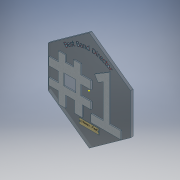
# Autodesk Inventor part: Trophy
Saved by Autodesk Inventor 2018 (Build 220112000, 112)
## iProperties
Created: 2019-03-04
Part Number: Trophy
Material: Generic
Document SubType Name: Modeling
Designer: This kid
Density: 1 g/cm^3
Appearance: Expanded Metal 01
Author: This kid
Autodesk Inventor part; units mm, degrees
(part 1 of 3)
ref_plane "YZ Plane" through (0, 0, 0) normal (1, 0, 0) x (0, 1, 0)
ref_plane "XZ Plane" through (0, 0, 0) normal (0, 1, 0) x (-1, 0, 0)
ref_plane "XY Plane" through (0, 0, 0) normal (0, 0, 1) x (1, 0, 0)
sketch "Sketch1" plane through (0, 0, 0) normal (0, 0, 1) x (1, 0, 0)
  line L0 (4871.8502, -2409.9611) -> (4871.8502, 2409.9611)
  line L1 (-4871.8502, 2409.9611) -> (-4871.8502, -2409.9611)
  line L2 (-4871.8502, 2409.9611) -> (0, 5903.7537)
  line L3 (0, 5903.7537) -> (4871.8502, 2409.9611)
  line L4 (-4871.8502, -2409.9611) -> (0, -5895.763)
  line L5 (0, -5895.763) -> (4871.8502, -2409.9611)
  point P0 (0, 0)
  constraints: 12 end point, 1 parallel
extrude "Extrusion1" add sketch "Sketch1" along normal blind 304.8
sketch "Sketch5" plane through (0, 0, 304.8) normal (0, 0, 1) x (1, 0, 0)
  line L0 (-1178.5841, -3968.2328) -> (1176.6192, -3968.2328)
  line L1 (1176.6192, -3968.2328) -> (1176.6192, -3311.2191)
  line L2 (1176.6192, -3311.2191) -> (-1178.5841, -3311.2191)
  line L3 (-1178.5841, -3311.2191) -> (-1178.5841, -3968.2328)
  line L4 (-1178.5841, -3968.2328) -> (1176.6192, -3311.2191) construction
  line L5 (1176.6192, -3968.2328) -> (-1178.5841, -3311.2191) construction
  point P0 (0, 0)
  point P1 (-0.9824, -3639.7259)
  constraints: 12 end point, 2 midpoint, 2 parallel, 1 horizontal, 1 perpendicular
extrude "Extrusion2" add sketch "Sketch5" along normal blind 25.4
sketch "Sketch6" plane through (0, 0, 330.2) normal (0, 0, 1) x (1, 0, 0)
  point P0 (0, 0)
sketch "Sketch7" plane through (0, 0, 330.2) normal (0, 0, 1) x (1, 0, 0)
  line L0 (-1178.5841, -3311.2191) -> (1176.6192, -3311.2191) construction
  line L1 (-0.9824, -3311.2191) -> (-0.9824, -3968.2328) construction
  line L2 (1176.6192, -3968.2328) -> (-1178.5841, -3968.2328) construction
  line L3 (-1178.5841, -3968.2328) -> (-1178.5841, -3311.2191) construction
  line L4 (-1178.5841, -3639.7259) -> (1176.6192, -3639.7259) construction
  line L5 (1176.6192, -3311.2191) -> (1176.6192, -3968.2328) construction
  line L6 (1176.6192, -3490.7913) -> (1021.494, -3490.7913) construction
  line L7 (-1178.5841, -3918.298) -> (-1023.4589, -3918.298) construction
  line L8 (-1101.0215, -3918.298) -> (-1101.0215, -3968.2328)
  line L9 (-1101.0215, -3311.2191) -> (-1101.0215, -3918.298)
  line L10 (1099.0566, -3490.7913) -> (1099.0566, -3311.2191)
  line L11 (1099.0566, -3968.2328) -> (1099.0566, -3490.7913)
  point P0 (0, 0)
  point P1 (-1023.4589, -3439.1683)
  point P2 (1110.7745, -3639.7259)
  point P3 (-1101.0215, -3639.7259)
  point P4 (1099.0566, -3639.7259)
  constraints: 16 end point, 12 point on line, 6 midpoint, 2 collinear, 2 perpendicular, 1 horizontal, 1 parallel
sketch "Sketch8" plane through (0, 0, 330.2) normal (0, 0, 1) x (1, 0, 0)
  line L0 (-1188.8601, -3420.1858) -> (1172.5443, -3420.1858) construction
  line L1 (1172.5443, -3420.1858) -> (1172.5443, -3747.7413) construction
  line L2 (1172.5443, -3747.7413) -> (-1188.8601, -3747.7413) construction
  line L3 (-1188.8601, -3747.7413) -> (-1188.8601, -3420.1858) construction
  point P0 (0, 0)
  constraints: 2 other
sketch "Sketch9" plane through (0, 0, 304.8) normal (0, 0, 1) x (1, 0, 0)
  arc A0 (3785.7257, 1434.029) -> (-2757.9123, 2963.4571) centre (0, 0) ccw construction
  spline S0 degree 2 poles (-2558.5983, 3341.4787) (-2534.2376, 3312.4793) (-2518.9668, 3249.4993) (-2525.0687, 3219.6418) knots 0 0 0 1 2 2 2
  spline S1 degree 2 poles (-2525.0687, 3219.6418) (-2532.8347, 3184.0851) (-2570.7728, 3127.4837) (-2610.4893, 3094.1201) knots 0 0 0 1 2 2 2
  line L0 (-2610.4893, 3094.1201) -> (-2722.0737, 3000.3842)
  line L1 (-2722.0737, 3000.3842) -> (-3048.8254, 3389.3537)
  line L2 (-3048.8254, 3389.3537) -> (-2945.7517, 3475.9402)
  spline S2 degree 2 poles (-2945.7517, 3475.9402) (-2904.1439, 3510.8926) (-2858.0347, 3540.4864) (-2830.384, 3545.9719) knots 0 0 0 1 2 2 2
  spline S3 degree 2 poles (-2830.384, 3545.9719) (-2799.9972, 3552.6805) (-2750.3185, 3532.5836) (-2729.6648, 3507.9972) knots 0 0 0 1 2 2 2
  spline S4 degree 2 poles (-2729.6648, 3507.9972) (-2706.628, 3480.5739) (-2699.0862, 3412.7141) (-2714.2914, 3378.9729) knots 0 0 0 1 2 2 2
  line L3 (-2714.2914, 3378.9729) -> (-2712.7027, 3377.0816)
  spline S5 degree 2 poles (-2712.7027, 3377.0816) (-2670.0858, 3396.7523) (-2589.8437, 3378.6735) (-2558.5983, 3341.4787) knots 0 0 0 1 2 2 2
  spline S6 degree 2 poles (-2610.6458, 3293.993) (-2629.1811, 3316.0577) (-2665.6207, 3333.835) (-2693.0066, 3328.0343) knots 0 0 0 1 2 2 2
  spline S7 degree 2 poles (-2693.0066, 3328.0343) (-2710.5956, 3324.0117) (-2742.7725, 3303.4335) (-2769.5654, 3280.9263) knots 0 0 0 1 2 2 2
  line L4 (-2769.5654, 3280.9263) -> (-2828.1945, 3231.6752)
  line L5 (-2828.1945, 3231.6752) -> (-2707.4499, 3087.9393)
  line L6 (-2707.4499, 3087.9393) -> (-2665.5269, 3123.1564)
  spline S8 degree 2 poles (-2665.5269, 3123.1564) (-2631.4842, 3151.7538) (-2597.694, 3190.8921) (-2591.0372, 3213.6888) knots 0 0 0 1 2 2 2
  spline S9 degree 2 poles (-2591.0372, 3213.6888) (-2585.2756, 3236.2711) (-2593.4344, 3273.5043) (-2610.6458, 3293.993) knots 0 0 0 1 2 2 2
  spline S10 degree 2 poles (-2777.4756, 3455.4681) (-2789.1264, 3469.3374) (-2816.0589, 3482.1975) (-2831.4918, 3479.4484) knots 0 0 0 1 2 2 2
  spline S11 degree 2 poles (-2831.4918, 3479.4484) (-2849.9256, 3475.7914) (-2883.1489, 3453.2589) (-2910.5722, 3430.2221) knots 0 0 0 1 2 2 2
  line L7 (-2910.5722, 3430.2221) -> (-2960.0602, 3388.6499)
  line L8 (-2960.0602, 3388.6499) -> (-2864.4708, 3274.859)
  line L9 (-2864.4708, 3274.859) -> (-2805.8417, 3324.1101)
  spline S12 degree 2 poles (-2805.8417, 3324.1101) (-2781.5705, 3344.499) (-2762.7968, 3368.872) (-2757.1234, 3387.0791) knots 0 0 0 1 2 2 2
  spline S13 degree 2 poles (-2757.1234, 3387.0791) (-2751.5003, 3404.7062) (-2762.1177, 3437.1859) (-2777.4756, 3455.4681) knots 0 0 0 1 2 2 2
  spline S14 degree 2 poles (-2266.0484, 3344.2576) (-2341.3465, 3292.4654) (-2482.1979, 3319.9967) (-2535.8564, 3398.0083) knots 0 0 0 1 2 2 2
  spline S15 degree 2 poles (-2535.8564, 3398.0083) (-2588.5818, 3474.6632) (-2570.7199, 3620.8553) (-2505.9363, 3665.4152) knots 0 0 0 1 2 2 2
  spline S16 degree 2 poles (-2505.9363, 3665.4152) (-2476.7668, 3685.4789) (-2419.9908, 3699.5485) (-2391.0061, 3693.0035) knots 0 0 0 1 2 2 2
  spline S17 degree 2 poles (-2391.0061, 3693.0035) (-2361.6823, 3686.6918) (-2308.0111, 3647.1619) (-2282.115, 3609.5129) knots 0 0 0 1 2 2 2
  line L10 (-2282.115, 3609.5129) -> (-2262.2847, 3580.6825)
  line L11 (-2262.2847, 3580.6825) -> (-2479.6996, 3431.1384)
  spline S18 degree 2 poles (-2479.6996, 3431.1384) (-2442.1386, 3376.5303) (-2347.2973, 3356.3247) (-2298.4553, 3389.9196) knots 0 0 0 1 2 2 2
  spline S19 degree 2 poles (-2298.4553, 3389.9196) (-2281.157, 3401.8178) (-2252.944, 3432.7155) (-2243.5761, 3448.1526) knots 0 0 0 1 2 2 2
  spline S20 degree 2 poles (-2243.5761, 3448.1526) (-2233.9965, 3464.7348) (-2222.4894, 3490.1374) (-2219.7778, 3499.997) knots 0 0 0 1 2 2 2
  line L12 (-2219.7778, 3499.997) -> (-2216.7252, 3502.0966)
  line L13 (-2216.7252, 3502.0966) -> (-2177.0645, 3444.4359)
  spline S21 degree 2 poles (-2177.0645, 3444.4359) (-2183.6561, 3434.4059) (-2204.0034, 3404.4216) (-2212.7575, 3393.9035) knots 0 0 0 1 2 2 2
  spline S22 degree 2 poles (-2212.7575, 3393.9035) (-2224.9877, 3378.9957) (-2247.0542, 3357.3223) (-2266.0484, 3344.2576) knots 0 0 0 1 2 2 2
  spline S23 degree 2 poles (-2341.6026, 3585.5837) (-2356.9788, 3606.4855) (-2387.2609, 3631.6244) (-2402.9727, 3636.3065) knots 0 0 0 1 2 2 2
  spline S24 degree 2 poles (-2402.9727, 3636.3065) (-2420.296, 3641.8788) (-2457.7584, 3634.5982) (-2479.1268, 3619.9004) knots 0 0 0 1 2 2 2
  spline S25 degree 2 poles (-2479.1268, 3619.9004) (-2500.156, 3605.4359) (-2521.0327, 3572.5893) (-2524.8445, 3551.98) knots 0 0 0 1 2 2 2
  spline S26 degree 2 poles (-2524.8445, 3551.98) (-2528.0838, 3531.2649) (-2519.5307, 3492.6791) (-2507.4621, 3471.5009) knots 0 0 0 1 2 2 2
  line L14 (-2507.4621, 3471.5009) -> (-2341.6026, 3585.5837)
  spline S27 degree 2 poles (-2007.8449, 3504.7842) (-2041.0949, 3485.8054) (-2108.8605, 3470.826) (-2133.5235, 3470.0209) knots 0 0 0 1 2 2 2
  line L15 (-2133.5235, 3470.0209) -> (-2169.2363, 3532.5882)
  line L16 (-2169.2363, 3532.5882) -> (-2166.3761, 3534.2208)
  spline S28 degree 2 poles (-2166.3761, 3534.2208) (-2155.9604, 3532.5818) (-2128.8991, 3530.0157) (-2108.5248, 3531.6909) knots 0 0 0 1 2 2 2
  spline S29 degree 2 poles (-2108.5248, 3531.6909) (-2090.7039, 3532.8568) (-2050.6672, 3542.437) (-2032.4333, 3552.8448) knots 0 0 0 1 2 2 2
  spline S30 degree 2 poles (-2032.4333, 3552.8448) (-2019.2048, 3560.3955) (-1992.2842, 3583.8197) (-1987.9907, 3592.9065) knots 0 0 0 1 2 2 2
  spline S31 degree 2 poles (-1987.9907, 3592.9065) (-1981.4998, 3605.6177) (-1980.9792, 3626.2972) (-1989.9585, 3642.0284) knots 0 0 0 1 2 2 2
  spline S32 degree 2 poles (-1989.9585, 3642.0284) (-2001.1825, 3661.6924) (-2034.2663, 3669.8271) (-2065.6733, 3660.9065) knots 0 0 0 1 2 2 2
  spline S33 degree 2 poles (-2065.6733, 3660.9065) (-2077.8276, 3657.287) (-2116.2317, 3644.8465) (-2133.1351, 3640.4123) knots 0 0 0 1 2 2 2
  spline S34 degree 2 poles (-2133.1351, 3640.4123) (-2177.3593, 3629.8639) (-2237.8033, 3656.0363) (-2256.374, 3688.5713) knots 0 0 0 1 2 2 2
  spline S35 degree 2 poles (-2256.374, 3688.5713) (-2282.0872, 3733.6198) (-2246.554, 3828.3214) (-2190.7798, 3860.1568) knots 0 0 0 1 2 2 2
  spline S36 degree 2 poles (-2190.7798, 3860.1568) (-2163.2502, 3875.8705) (-2099.7211, 3894.1198) (-2074.854, 3894.5674) knots 0 0 0 1 2 2 2
  line L17 (-2074.854, 3894.5674) -> (-2040.7738, 3834.8604)
  line L18 (-2040.7738, 3834.8604) -> (-2043.634, 3833.2278)
  spline S37 degree 2 poles (-2043.634, 3833.2278) (-2074.8812, 3838.1447) (-2138.3042, 3828.014) (-2165.1188, 3812.7085) knots 0 0 0 1 2 2 2
  spline S38 degree 2 poles (-2165.1188, 3812.7085) (-2192.6484, 3796.9949) (-2217.2815, 3752.1239) (-2204.0167, 3728.8846) knots 0 0 0 1 2 2 2
  spline S39 degree 2 poles (-2204.0167, 3728.8846) (-2191.9764, 3707.7905) (-2157.82, 3700.268) (-2129.1198, 3708.1177) knots 0 0 0 1 2 2 2
  spline S40 degree 2 poles (-2129.1198, 3708.1177) (-2115.1272, 3711.8384) (-2080.7065, 3722.9532) (-2061.6579, 3728.6118) knots 0 0 0 1 2 2 2
  spline S41 degree 2 poles (-2061.6579, 3728.6118) (-2019.8843, 3740.1316) (-1958.4167, 3718.8095) (-1937.3972, 3681.9842) knots 0 0 0 1 2 2 2
  spline S42 degree 2 poles (-1937.3972, 3681.9842) (-1925.1528, 3660.5325) (-1920.3248, 3613.0432) (-1928.8122, 3589.7122) knots 0 0 0 1 2 2 2
  spline S43 degree 2 poles (-1928.8122, 3589.7122) (-1937.964, 3565.054) (-1973.8798, 3524.1712) (-2007.8449, 3504.7842) knots 0 0 0 1 2 2 2
  spline S44 degree 2 poles (-1722.0451, 3655.7889) (-1769.0922, 3632.9858) (-1848.1015, 3661.0251) (-1876.2911, 3719.1856) knots 0 0 0 1 2 2 2
  line L19 (-1876.2911, 3719.1856) -> (-1968.4012, 3909.2262)
  line L20 (-1968.4012, 3909.2262) -> (-2007.2984, 3890.3733)
  line L21 (-2007.2984, 3890.3733) -> (-2030.4605, 3938.1613)
  line L22 (-2030.4605, 3938.1613) -> (-1991.5633, 3957.0142)
  line L23 (-1991.5633, 3957.0142) -> (-2039.3241, 4055.5538)
  line L24 (-2039.3241, 4055.5538) -> (-1981.534, 4083.5639)
  line L25 (-1981.534, 4083.5639) -> (-1933.7732, 3985.0243)
  line L26 (-1933.7732, 3985.0243) -> (-1827.4542, 4036.5556)
  line L27 (-1827.4542, 4036.5556) -> (-1804.292, 3988.7677)
  line L28 (-1804.292, 3988.7677) -> (-1910.611, 3937.2363)
  line L29 (-1910.611, 3937.2363) -> (-1831.4287, 3773.8681)
  spline S45 degree 2 poles (-1831.4287, 3773.8681) (-1818.8601, 3747.9366) (-1803.1824, 3720.3098) (-1790.9595, 3711.1373) knots 0 0 0 1 2 2 2
  spline S46 degree 2 poles (-1790.9595, 3711.1373) (-1780.5662, 3702.908) (-1752.0209, 3703.4767) (-1732.0166, 3713.1725) knots 0 0 0 1 2 2 2
  spline S47 degree 2 poles (-1732.0166, 3713.1725) (-1717.9396, 3719.9955) (-1695.7673, 3741.264) (-1691.097, 3746.73) knots 0 0 0 1 2 2 2
  line L30 (-1691.097, 3746.73) -> (-1687.763, 3748.3459)
  line L31 (-1687.763, 3748.3459) -> (-1662.6257, 3696.483)
  spline S48 degree 2 poles (-1662.6257, 3696.483) (-1676.7709, 3684.1373) (-1707.5976, 3662.7914) (-1722.0451, 3655.7889) knots 0 0 0 1 2 2 2
  spline S49 degree 2 poles (-1132.9212, 4053.1956) (-1121.0879, 4017.2181) (-1130.3262, 3953.0751) (-1147.0909, 3927.6262) knots 0 0 0 1 2 2 2
  spline S50 degree 2 poles (-1147.0909, 3927.6262) (-1167.5195, 3897.5053) (-1223.7813, 3859.0655) (-1273.0548, 3842.8589) knots 0 0 0 1 2 2 2
  line L32 (-1273.0548, 3842.8589) -> (-1411.4899, 3797.3262)
  line L33 (-1411.4899, 3797.3262) -> (-1570.2112, 4279.8939)
  line L34 (-1570.2112, 4279.8939) -> (-1442.3347, 4321.9537)
  spline S51 degree 2 poles (-1442.3347, 4321.9537) (-1390.7148, 4338.932) (-1336.9083, 4349.2623) (-1309.2002, 4344.0747) knots 0 0 0 1 2 2 2
  spline S52 degree 2 poles (-1309.2002, 4344.0747) (-1278.4973, 4339.0054) (-1239.851, 4301.8796) (-1229.8184, 4271.3769) knots 0 0 0 1 2 2 2
  spline S53 degree 2 poles (-1229.8184, 4271.3769) (-1218.6282, 4237.3547) (-1236.8556, 4171.5551) (-1263.5151, 4145.8853) knots 0 0 0 1 2 2 2
  line L35 (-1263.5151, 4145.8853) -> (-1262.7434, 4143.539)
  spline S54 degree 2 poles (-1262.7434, 4143.539) (-1215.8681, 4145.9557) (-1148.0988, 4099.3407) (-1132.9212, 4053.1956) knots 0 0 0 1 2 2 2
  spline S55 degree 2 poles (-1198.8921, 4028.4636) (-1207.8957, 4055.8378) (-1235.1142, 4085.8882) (-1262.6937, 4090.6847) knots 0 0 0 1 2 2 2
  spline S56 degree 2 poles (-1262.6937, 4090.6847) (-1280.5175, 4093.4896) (-1318.0385, 4086.349) (-1351.2786, 4075.416) knots 0 0 0 1 2 2 2
  line L36 (-1351.2786, 4075.416) -> (-1424.0157, 4051.492)
  line L37 (-1424.0157, 4051.492) -> (-1365.3634, 3873.1688)
  line L38 (-1365.3634, 3873.1688) -> (-1313.3525, 3890.2757)
  spline S57 degree 2 poles (-1313.3525, 3890.2757) (-1271.118, 3904.1671) (-1225.1991, 3927.9376) (-1210.5442, 3946.6254) knots 0 0 0 1 2 2 2
  spline S58 degree 2 poles (-1210.5442, 3946.6254) (-1196.8, 3965.447) (-1190.5316, 4003.0447) (-1198.8921, 4028.4636) knots 0 0 0 1 2 2 2
  spline S59 degree 2 poles (-1293.7313, 4240.3879) (-1299.3907, 4257.5946) (-1319.6116, 4279.5458) (-1334.9604, 4282.7314) knots 0 0 0 1 2 2 2
  spline S60 degree 2 poles (-1334.9604, 4282.7314) (-1353.4325, 4286.1898) (-1392.6516, 4277.6239) (-1426.6738, 4266.4336) knots 0 0 0 1 2 2 2
  line L39 (-1426.6738, 4266.4336) -> (-1488.0701, 4246.2398)
  line L40 (-1488.0701, 4246.2398) -> (-1441.6371, 4105.0672)
  line L41 (-1441.6371, 4105.0672) -> (-1368.9, 4128.9912)
  spline S61 degree 2 poles (-1368.9, 4128.9912) (-1338.7884, 4138.8952) (-1312.299, 4154.5416) (-1300.2633, 4169.3344) knots 0 0 0 1 2 2 2
  spline S62 degree 2 poles (-1300.2633, 4169.3344) (-1288.49, 4183.6076) (-1286.2711, 4217.7065) (-1293.7313, 4240.3879) knots 0 0 0 1 2 2 2
  spline S63 degree 2 poles (-825.2961, 4005.1241) (-831.6592, 3997.7819) (-852.8354, 3971.9091) (-863.5255, 3963.1697) knots 0 0 0 1 2 2 2
  spline S64 degree 2 poles (-863.5255, 3963.1697) (-877.9995, 3950.6234) (-906.8404, 3934.4169) (-934.952, 3928.0807) knots 0 0 0 1 2 2 2
  spline S65 degree 2 poles (-934.952, 3928.0807) (-957.8429, 3922.9212) (-1003.0994, 3930.8665) (-1022.2918, 3942.9985) knots 0 0 0 1 2 2 2
  spline S66 degree 2 poles (-1022.2918, 3942.9985) (-1040.5904, 3954.91) (-1068.8001, 3995.8153) (-1074.4122, 4020.7142) knots 0 0 0 1 2 2 2
  spline S67 degree 2 poles (-1074.4122, 4020.7142) (-1083.1018, 4059.2673) (-1062.883, 4121.2161) (-1031.0728, 4144.8438) knots 0 0 0 1 2 2 2
  spline S68 degree 2 poles (-1031.0728, 4144.8438) (-1003.007, 4166.3615) (-920.3129, 4196.3942) (-871.5504, 4210.339) knots 0 0 0 1 2 2 2
  line L42 (-871.5504, 4210.339) -> (-874.2659, 4222.3868)
  spline S69 degree 2 poles (-874.2659, 4222.3868) (-879.1539, 4244.0729) (-898.4711, 4267.9927) (-912.2388, 4272.9075) knots 0 0 0 1 2 2 2
  spline S70 degree 2 poles (-912.2388, 4272.9075) (-926.0065, 4277.8223) (-961.6298, 4274.8569) (-980.1032, 4270.6932) knots 0 0 0 1 2 2 2
  spline S71 degree 2 poles (-980.1032, 4270.6932) (-1001.7893, 4265.8052) (-1057.5256, 4239.7387) (-1084.0359, 4220.6815) knots 0 0 0 1 2 2 2
  line L43 (-1084.0359, 4220.6815) -> (-1087.6503, 4219.8668)
  line L44 (-1087.6503, 4219.8668) -> (-1102.0425, 4283.7204)
  spline S72 degree 2 poles (-1102.0425, 4283.7204) (-1085.8602, 4292.4318) (-1023.9189, 4319.0529) (-992.193, 4326.2037) knots 0 0 0 1 2 2 2
  spline S73 degree 2 poles (-992.193, 4326.2037) (-953.6399, 4334.8934) (-898.3154, 4334.7033) (-873.9023, 4323.748) knots 0 0 0 1 2 2 2
  spline S74 degree 2 poles (-873.9023, 4323.748) (-849.9814, 4313.1038) (-818.949, 4269.0367) (-811.0741, 4234.0979) knots 0 0 0 1 2 2 2
  line L45 (-811.0741, 4234.0979) -> (-753.7767, 3979.8885)
  line L46 (-753.7767, 3979.8885) -> (-816.4254, 3965.7678)
  line L47 (-816.4254, 3965.7678) -> (-825.2961, 4005.1241)
  line L48 (-837.0634, 4057.3314) -> (-860.3263, 4160.5412)
  spline S75 degree 2 poles (-860.3263, 4160.5412) (-882.363, 4153.4643) (-948.6937, 4131.3398) (-968.53, 4120.1169) knots 0 0 0 1 2 2 2
  spline S76 degree 2 poles (-968.53, 4120.1169) (-991.709, 4106.8745) (-1017.0873, 4067.8166) (-1010.7511, 4039.705) knots 0 0 0 1 2 2 2
  spline S77 degree 2 poles (-1010.7511, 4039.705) (-1003.5097, 4007.5774) (-960.0343, 3983.1948) (-925.4972, 3990.9793) knots 0 0 0 1 2 2 2
  spline S78 degree 2 poles (-925.4972, 3990.9793) (-896.1808, 3997.587) (-853.692, 4033.7496) (-837.0634, 4057.3314) knots 0 0 0 1 2 2 2
  line L49 (-368.3427, 4034.2667) -> (-432.0348, 4026.0464)
  line L50 (-432.0348, 4026.0464) -> (-459.8575, 4241.6198)
  spline S79 degree 2 poles (-459.8575, 4241.6198) (-463.23, 4267.7499) (-473.9258, 4312.0286) (-483.0138, 4324.5535) knots 0 0 0 1 2 2 2
  spline S80 degree 2 poles (-483.0138, 4324.5535) (-492.6155, 4337.8422) (-522.1704, 4348.1406) (-545.8508, 4345.0843) knots 0 0 0 1 2 2 2
  spline S81 degree 2 poles (-545.8508, 4345.0843) (-569.5312, 4342.028) (-616.4829, 4310.233) (-637.9369, 4286.7099) knots 0 0 0 1 2 2 2
  line L51 (-637.9369, 4286.7099) -> (-601.4722, 4004.1781)
  line L52 (-601.4722, 4004.1781) -> (-665.1643, 3995.9577)
  line L53 (-665.1643, 3995.9577) -> (-713.9596, 4374.0277)
  line L54 (-713.9596, 4374.0277) -> (-650.2674, 4382.2481)
  line L55 (-650.2674, 4382.2481) -> (-644.8399, 4340.1949)
  spline S82 degree 2 poles (-644.8399, 4340.1949) (-619.5798, 4369.6054) (-567.9395, 4403.6658) (-536.91, 4407.6706) knots 0 0 0 1 2 2 2
  spline S83 degree 2 poles (-536.91, 4407.6706) (-481.3835, 4414.8371) (-409.0229, 4349.4611) (-400.0121, 4279.6448) knots 0 0 0 1 2 2 2
  line L56 (-400.0121, 4279.6448) -> (-368.3427, 4034.2667)
  line L57 (14.388, 4050.8554) -> (-49.7982, 4048.76)
  line L58 (-49.7982, 4048.76) -> (-51.0608, 4087.4363)
  spline S84 degree 2 poles (-51.0608, 4087.4363) (-65.4701, 4074.6092) (-86.7396, 4057.4393) (-101.3235, 4049.9611) knots 0 0 0 1 2 2 2
  spline S85 degree 2 poles (-101.3235, 4049.9611) (-114.6864, 4042.9346) (-143.6711, 4034.9863) (-163.0092, 4034.355) knots 0 0 0 1 2 2 2
  spline S86 degree 2 poles (-163.0092, 4034.355) (-194.2794, 4033.3341) (-247.7913, 4057.5362) (-267.1259, 4082.0302) knots 0 0 0 1 2 2 2
  spline S87 degree 2 poles (-267.1259, 4082.0302) (-286.4605, 4106.5242) (-309.4508, 4179.9136) (-311.0224, 4228.0533) knots 0 0 0 1 2 2 2
  spline S88 degree 2 poles (-311.0224, 4228.0533) (-312.6611, 4278.2502) (-289.1307, 4352.3346) (-267.4009, 4380.6405) knots 0 0 0 1 2 2 2
  spline S89 degree 2 poles (-267.4009, 4380.6405) (-247.2229, 4406.0126) (-189.3123, 4436.3234) (-156.8078, 4437.3846) knots 0 0 0 1 2 2 2
  spline S90 degree 2 poles (-156.8078, 4437.3846) (-128.4177, 4438.3114) (-85.6219, 4426.9399) (-61.7394, 4414.5392) knots 0 0 0 1 2 2 2
  line L59 (-61.7394, 4414.5392) -> (-67.1123, 4579.1192)
  line L60 (-67.1123, 4579.1192) -> (-2.9261, 4581.2147)
  line L61 (-2.9261, 4581.2147) -> (14.388, 4050.8554)
  line L62 (-52.8205, 4141.3363) -> (-60.0067, 4361.4621)
  spline S91 degree 2 poles (-60.0067, 4361.4621) (-84.2469, 4372.2036) (-122.3824, 4379.6083) (-144.1892, 4378.8964) knots 0 0 0 1 2 2 2
  spline S92 degree 2 poles (-144.1892, 4378.8964) (-193.5633, 4377.2846) (-247.1027, 4301.3968) (-244.8192, 4231.4502) knots 0 0 0 1 2 2 2
  spline S93 degree 2 poles (-244.8192, 4231.4502) (-242.6163, 4163.9724) (-197.5017, 4094.1885) (-150.185, 4095.7332) knots 0 0 0 1 2 2 2
  spline S94 degree 2 poles (-150.185, 4095.7332) (-125.0865, 4096.5525) (-74.8189, 4121.2593) (-52.8205, 4141.3363) knots 0 0 0 1 2 2 2
  spline S95 degree 2 poles (759.7655, 4239.6528) (750.9285, 4170.6442) (680.7638, 4066.7408) (629.8313, 4041.7206) knots 0 0 0 1 2 2 2
  spline S96 degree 2 poles (629.8313, 4041.7206) (588.3627, 4022.5441) (507.4625, 4016.3026) (446.2122, 4024.146) knots 0 0 0 1 2 2 2
  line L63 (446.2122, 4024.146) -> (330.2451, 4038.9963)
  line L64 (330.2451, 4038.9963) -> (394.7705, 4542.8816)
  line L65 (394.7705, 4542.8816) -> (509.5126, 4528.1883)
  spline S97 degree 2 poles (509.5126, 4528.1883) (580.5629, 4519.0899) (658.6942, 4487.5031) (684.8723, 4465.0594) knots 0 0 0 1 2 2 2
  spline S98 degree 2 poles (684.8723, 4465.0594) (729.3333, 4426.5785) (769.1776, 4313.1531) (759.7655, 4239.6528) knots 0 0 0 1 2 2 2
  spline S99 degree 2 poles (690.0448, 4249.411) (697.4699, 4307.3946) (669.5966, 4394.3851) (634.602, 4422.5232) knots 0 0 0 1 2 2 2
  spline S100 degree 2 poles (634.602, 4422.5232) (609.6911, 4441.8993) (550.6794, 4463.9822) (505.3542, 4469.7864) knots 0 0 0 1 2 2 2
  line L66 (505.3542, 4469.7864) -> (454.3123, 4476.3226)
  line L67 (454.3123, 4476.3226) -> (404.6372, 4088.4043)
  line L68 (404.6372, 4088.4043) -> (455.679, 4081.8681)
  spline S101 degree 2 poles (455.679, 4081.8681) (500.1876, 4076.1686) (569.393, 4081.8325) (599.209, 4097.5208) knots 0 0 0 1 2 2 2
  spline S102 degree 2 poles (599.209, 4097.5208) (637.3586, 4116.7074) (682.515, 4190.6108) (690.0448, 4249.411) knots 0 0 0 1 2 2 2
  line L69 (857.6796, 3956.4599) -> (794.811, 3969.5673)
  line L70 (794.811, 3969.5673) -> (872.6153, 4342.7488)
  line L71 (872.6153, 4342.7488) -> (935.4839, 4329.6414)
  line L72 (935.4839, 4329.6414) -> (857.6796, 3956.4599)
  line L73 (952.8563, 4390.7797) -> (881.5246, 4405.6516)
  line L74 (881.5246, 4405.6516) -> (895.1362, 4470.9382)
  line L75 (895.1362, 4470.9382) -> (966.4678, 4456.0663)
  line L76 (966.4678, 4456.0663) -> (952.8563, 4390.7797)
  line L77 (1224.4433, 4187.0481) -> (1221.2576, 4187.8832)
  spline S103 degree 2 poles (1221.2576, 4187.8832) (1214.6117, 4191.7533) (1199.2901, 4196.6209) (1188.5383, 4199.4395) knots 0 0 0 1 2 2 2
  spline S104 degree 2 poles (1188.5383, 4199.4395) (1163.4509, 4206.0161) (1108.3309, 4197.0587) (1080.3938, 4181.4011) knots 0 0 0 1 2 2 2
  line L78 (1080.3938, 4181.4011) -> (1011.8093, 3919.7745)
  line L79 (1011.8093, 3919.7745) -> (949.6879, 3936.0594)
  line L80 (949.6879, 3936.0594) -> (1046.3535, 4304.8055)
  line L81 (1046.3535, 4304.8055) -> (1108.4748, 4288.5206)
  line L82 (1108.4748, 4288.5206) -> (1094.069, 4233.5671)
  spline S105 degree 2 poles (1094.069, 4233.5671) (1135.8508, 4254.9581) (1192.8962, 4266.3898) (1216.789, 4260.1264) knots 0 0 0 1 2 2 2
  spline S106 degree 2 poles (1216.789, 4260.1264) (1226.3462, 4257.621) (1235.6945, 4254.3192) (1241.3545, 4251.5587) knots 0 0 0 1 2 2 2
  line L83 (1241.3545, 4251.5587) -> (1224.4433, 4187.0481)
  spline S107 degree 2 poles (1346.5719, 3808.6452) (1260.1975, 3838.5068) (1198.7569, 3968.2069) (1229.6946, 4057.6939) knots 0 0 0 1 2 2 2
  spline S108 degree 2 poles (1229.6946, 4057.6939) (1260.0942, 4145.6245) (1388.3537, 4218.017) (1462.6668, 4192.3253) knots 0 0 0 1 2 2 2
  spline S109 degree 2 poles (1462.6668, 4192.3253) (1496.1271, 4180.7573) (1541.1484, 4143.4136) (1553.0838, 4116.2016) knots 0 0 0 1 2 2 2
  spline S110 degree 2 poles (1553.0838, 4116.2016) (1565.4084, 4088.8551) (1565.4491, 4022.1978) (1550.5183, 3979.0106) knots 0 0 0 1 2 2 2
  line L84 (1550.5183, 3979.0106) -> (1539.0848, 3945.9393)
  line L85 (1539.0848, 3945.9393) -> (1289.6886, 4032.1612)
  spline S111 degree 2 poles (1289.6886, 4032.1612) (1268.0322, 3969.5204) (1308.0607, 3881.1979) (1364.0873, 3861.8282) knots 0 0 0 1 2 2 2
  spline S112 degree 2 poles (1364.0873, 3861.8282) (1383.93, 3854.9681) (1425.5421, 3850.6002) (1443.5262, 3852.2231) knots 0 0 0 1 2 2 2
  spline S113 degree 2 poles (1443.5262, 3852.2231) (1462.5576, 3854.355) (1489.8317, 3860.171) (1499.3763, 3863.8404) knots 0 0 0 1 2 2 2
  line L86 (1499.3763, 3863.8404) -> (1502.878, 3862.6298)
  line L87 (1502.878, 3862.6298) -> (1480.011, 3796.4873)
  spline S114 degree 2 poles (1480.011, 3796.4873) (1468.0264, 3795.8393) (1431.818, 3794.4189) (1418.157, 3795.2216) knots 0 0 0 1 2 2 2
  spline S115 degree 2 poles (1418.157, 3795.2216) (1398.9001, 3796.2167) (1368.36, 3801.1126) (1346.5719, 3808.6452) knots 0 0 0 1 2 2 2
  spline S116 degree 2 poles (1495.9525, 4012.6848) (1503.6485, 4037.4655) (1505.9077, 4076.7576) (1500.3507, 4092.1816) knots 0 0 0 1 2 2 2
  spline S117 degree 2 poles (1500.3507, 4092.1816) (1494.5536, 4109.431) (1466.4593, 4135.2602) (1441.9477, 4143.7345) knots 0 0 0 1 2 2 2
  spline S118 degree 2 poles (1441.9477, 4143.7345) (1417.8251, 4152.0742) (1378.9988, 4149.381) (1360.1497, 4140.2167) knots 0 0 0 1 2 2 2
  spline S119 degree 2 poles (1360.1497, 4140.2167) (1341.5552, 4130.5289) (1315.577, 4100.7438) (1305.6955, 4078.461) knots 0 0 0 1 2 2 2
  line L88 (1305.6955, 4078.461) -> (1495.9525, 4012.6848)
  spline S120 degree 2 poles (1673.5636, 3676.7895) (1637.4463, 3692.833) (1587.4871, 3741.6021) (1576.0697, 3773.7012) knots 0 0 0 1 2 2 2
  spline S121 degree 2 poles (1576.0697, 3773.7012) (1564.4851, 3805.4241) (1571.1989, 3884.4249) (1591.5874, 3930.324) knots 0 0 0 1 2 2 2
  spline S122 degree 2 poles (1591.5874, 3930.324) (1611.976, 3976.223) (1666.1777, 4032.3277) (1696.8971, 4045.7094) knots 0 0 0 1 2 2 2
  spline S123 degree 2 poles (1696.8971, 4045.7094) (1727.7835, 4059.4674) (1799.9704, 4056.6813) (1835.3353, 4040.9721) knots 0 0 0 1 2 2 2
  spline S124 degree 2 poles (1835.3353, 4040.9721) (1863.9281, 4028.271) (1910.1655, 3988.3625) (1926.1783, 3968.6367) knots 0 0 0 1 2 2 2
  line L89 (1926.1783, 3968.6367) -> (1896.9324, 3902.7979)
  line L90 (1896.9324, 3902.7979) -> (1893.5464, 3904.302)
  spline S125 degree 2 poles (1893.5464, 3904.302) (1889.4903, 3912.4101) (1875.9431, 3934.6443) (1865.1981, 3947.976) knots 0 0 0 1 2 2 2
  spline S126 degree 2 poles (1865.1981, 3947.976) (1855.4567, 3959.5105) (1826.5272, 3983.6225) (1811.4784, 3990.3073) knots 0 0 0 1 2 2 2
  spline S127 degree 2 poles (1811.4784, 3990.3073) (1765.9555, 4010.5288) (1680.0681, 3966.2468) (1652.1591, 3903.4177) knots 0 0 0 1 2 2 2
  spline S128 degree 2 poles (1652.1591, 3903.4177) (1624.9187, 3842.0936) (1647.7593, 3749.5141) (1695.1632, 3728.457) knots 0 0 0 1 2 2 2
  spline S129 degree 2 poles (1695.1632, 3728.457) (1723.756, 3715.7559) (1786.2032, 3716.3954) (1814.3318, 3725.9729) knots 0 0 0 1 2 2 2
  line L91 (1814.3318, 3725.9729) -> (1817.7178, 3724.4689)
  line L92 (1817.7178, 3724.4689) -> (1788.4718, 3658.6301)
  spline S130 degree 2 poles (1788.4718, 3658.6301) (1777.9804, 3658.3354) (1746.4642, 3658.3709) (1734.7602, 3660.4167) knots 0 0 0 1 2 2 2
  spline S131 degree 2 poles (1734.7602, 3660.4167) (1717.7059, 3662.5868) (1691.9985, 3668.6007) (1673.5636, 3676.7895) knots 0 0 0 1 2 2 2
  spline S132 degree 2 poles (1929.5556, 3550.6404) (1883.3442, 3575.0927) (1859.2289, 3655.3867) (1889.4574, 3712.5141) knots 0 0 0 1 2 2 2
  line L93 (1889.4574, 3712.5141) -> (1988.2294, 3899.179)
  line L94 (1988.2294, 3899.179) -> (1950.0231, 3919.3955)
  line L95 (1950.0231, 3919.3955) -> (1974.8605, 3966.3346)
  line L96 (1974.8605, 3966.3346) -> (2013.0668, 3946.1181)
  line L97 (2013.0668, 3946.1181) -> (2064.2819, 4042.9073)
  line L98 (2064.2819, 4042.9073) -> (2121.0455, 4012.8714)
  line L99 (2121.0455, 4012.8714) -> (2069.8304, 3916.0822)
  line L100 (2069.8304, 3916.0822) -> (2174.2608, 3860.8238)
  line L101 (2174.2608, 3860.8238) -> (2149.4234, 3813.8847)
  line L102 (2149.4234, 3813.8847) -> (2044.993, 3869.1431)
  line L103 (2044.993, 3869.1431) -> (1960.0837, 3708.6768)
  spline S133 degree 2 poles (1960.0837, 3708.6768) (1946.606, 3683.2059) (1933.5999, 3654.2253) (1933.432, 3638.9445) knots 0 0 0 1 2 2 2
  spline S134 degree 2 poles (1933.432, 3638.9445) (1932.9425, 3625.6967) (1950.2827, 3603.0146) (1969.9316, 3592.6176) knots 0 0 0 1 2 2 2
  spline S135 degree 2 poles (1969.9316, 3592.6176) (1983.7586, 3585.3011) (2014.0217, 3579.9999) (2021.1914, 3579.4664) knots 0 0 0 1 2 2 2
  line L104 (2021.1914, 3579.4664) -> (2024.4662, 3577.7336)
  line L105 (2024.4662, 3577.7336) -> (1997.5109, 3526.7919)
  spline S136 degree 2 poles (1997.5109, 3526.7919) (1979.1902, 3530.8971) (1943.7464, 3543.1314) (1929.5556, 3550.6404) knots 0 0 0 1 2 2 2
  spline S137 degree 2 poles (2404.0697, 3495.3) (2352.7081, 3413.8041) (2218.3758, 3374.3805) (2152.9004, 3415.6453) knots 0 0 0 1 2 2 2
  spline S138 degree 2 poles (2152.9004, 3415.6453) (2085.6837, 3458.0076) (2066.4422, 3598.1116) (2116.0478, 3676.8213) knots 0 0 0 1 2 2 2
  spline S139 degree 2 poles (2116.0478, 3676.8213) (2166.9703, 3757.6207) (2302.7865, 3797.0823) (2367.5653, 3756.2565) knots 0 0 0 1 2 2 2
  spline S140 degree 2 poles (2367.5653, 3756.2565) (2433.0406, 3714.9916) (2455.2117, 3576.4476) (2404.0697, 3495.3) knots 0 0 0 1 2 2 2
  spline S141 degree 2 poles (2347.9977, 3530.6385) (2387.5066, 3593.3276) (2380.2942, 3683.0291) (2338.1531, 3709.5879) knots 0 0 0 1 2 2 2
  spline S142 degree 2 poles (2338.1531, 3709.5879) (2296.0121, 3736.1466) (2211.6286, 3704.172) (2172.1198, 3641.4828) knots 0 0 0 1 2 2 2
  spline S143 degree 2 poles (2172.1198, 3641.4828) (2133.7084, 3580.535) (2140.1715, 3488.8727) (2182.3126, 3462.3139) knots 0 0 0 1 2 2 2
  spline S144 degree 2 poles (2182.3126, 3462.3139) (2224.1054, 3435.9747) (2308.9278, 3468.6459) (2347.9977, 3530.6385) knots 0 0 0 1 2 2 2
  line L106 (2703.4596, 3423.7318) -> (2700.8185, 3425.6992)
  spline S145 degree 2 poles (2700.8185, 3425.6992) (2696.1057, 3431.7767) (2683.7223, 3442.0283) (2674.8087, 3448.6684) knots 0 0 0 1 2 2 2
  spline S146 degree 2 poles (2674.8087, 3448.6684) (2654.0102, 3464.1621) (2599.5472, 3476.5002) (2567.7793, 3472.4451) knots 0 0 0 1 2 2 2
  line L107 (2567.7793, 3472.4451) -> (2406.2021, 3255.5463)
  line L108 (2406.2021, 3255.5463) -> (2354.701, 3293.9117)
  line L109 (2354.701, 3293.9117) -> (2582.4339, 3599.6168)
  line L110 (2582.4339, 3599.6168) -> (2633.9349, 3561.2515)
  line L111 (2633.9349, 3561.2515) -> (2599.9963, 3515.6928)
  spline S147 degree 2 poles (2599.9963, 3515.6928) (2646.7487, 3519.8789) (2703.9236, 3509.1139) (2723.7317, 3494.358) knots 0 0 0 1 2 2 2
  spline S148 degree 2 poles (2723.7317, 3494.358) (2731.6549, 3488.4557) (2739.0863, 3481.893) (2743.3006, 3477.2136) knots 0 0 0 1 2 2 2
  line L112 (2743.3006, 3477.2136) -> (2703.4596, 3423.7318)
  point P0 (-3071.9487, 0)
  constraints: 2 point on circle, 1 centre point, 1 coincident, 2 other
hole "Hole2" at (-1101.0215, -3639.7259, 330.2) at (1099.0566, -3639.7259, 330.2) direction (0, 0, -1) diameter 4.9784 end through all countersink diameter 127 countersink angle 82 thread size "1/4-20 UNC" class "2B" standard "ANSI Unified Screw Threads"
sketch "Sketch10" plane through (0, 0, 330.2) normal (0, 0, 1) x (1, 0, 0)
  circle A0 centre (-1101.0215, -3639.7259) radius 2.4892 projected
  circle A1 centre (1099.3793, -3639.7259) radius 76.2
  circle A2 centre (-1101.0215, -3639.7259) radius 76.2
  point P0 (0, 0)
  dimension "d20" = 152.4
  dimension "d21" = 152.4
  constraints: 2 centre point, 1 coincident
  measures "d20" diameter of A1
  measures "d21" diameter of A2
extrude "Extrusion3" cut sketch "Sketch10" against normal blind 25.4
sketch "Sketch11" plane through (0, 0, 0) normal (0, 0, -1) x (-1, 0, 0)
  point P0 (0, 0)
extrude "Extrusion4" cut sketch "Sketch9" against normal blind 25.4
sketch "Sketch12" plane through (0, 0, 304.8) normal (0, 0, 1) x (1, 0, 0)
  line L0 (-3577.2096, 1436.9902) -> (2286.4087, -871.706)
  line L1 (-3577.2096, 1436.9902) -> (2221.8605, -1002.6019)
  line L2 (-4074.0857, 1652.9348) -> (2768.1418, -1149.8418) construction
  line L3 (1396.0365, -655.1886) -> (1419.6789, -597.4719) construction
  line L4 (1443.3213, -539.7553) -> (1419.6789, -597.4719) construction
  line L5 (2460.6287, -1152.1397) -> (2767.6599, -1395.4628)
  line L6 (2550.6115, -932.4707) -> (2940.1119, -974.4674)
  arc A0 (2767.6599, -1395.4628) -> (2940.1119, -974.4674) centre (2900.3058, -1203.98) ccw
  arc A1 (2286.4087, -871.706) -> (2550.6115, -932.4707) centre (2673.3643, 206.0087) ccw
  arc A2 (2460.6287, -1152.1397) -> (2221.8605, -1002.6019) centre (1881.7725, -1811.0134) ccw
  constraints: 14 end point, 6 point on circle, 3 centre point, 3 point on line, 2 symmetric about line, 2 tangent, 1 collinear, 1 perpendicular
sketch "Sketch14" plane through (0, 0, 304.8) normal (0, 0, 1) x (1, 0, 0)
  arc A0 (57.6983, 1248.2769) -> (-209.5648, 1248.2771) centre (-75.9333, 1226.17) ccw
  arc A1 (-1492.3011, 1043.103) -> (-209.5648, 904.9842) centre (-370.5499, 5435.4559) ccw
  arc A2 (-209.5648, 904.9842) -> (57.6983, 904.9842) centre (-75.9333, 910.7923) ccw
  arc A3 (57.6983, 904.9842) -> (1344.037, 1069.6986) centre (239.9233, 4587.0916) ccw
  arc A4 (1344.037, 1069.6986) -> (1610.4923, 1148.3247) centre (1476.8524, 1110.4085) ccw
  arc A5 (57.6983, 1248.2769) -> (1344.037, 1384.9498) centre (-63.8801, 8514.2713) ccw
  arc A6 (1610.4923, 1442.784) -> (1344.037, 1384.9498) centre (1482.0447, 1391.8442) ccw
  arc A7 (1610.4923, 1442.784) -> (1903.0093, 1658.484) centre (1392.8224, 2044.1679) ccw
  arc A8 (1610.4923, 1148.3247) -> (1925.3848, 1422.0781) centre (1428.0474, 1676.1709) ccw
  arc A9 (-2082.4405, 1731.2909) -> (-1787.8938, 1459.2764) centre (-1095.8709, 2504.1026) ccw
  arc A10 (-1787.8938, 1129.3874) -> (-1492.3011, 1043.103) centre (-1628.5464, 1125.8168) ccw
  arc A11 (-2098.725, 1402.2239) -> (-1787.8938, 1129.3874) centre (-1097.8602, 2228.9905) ccw
  line L0 (-75.9333, 777.0346) -> (-75.9333, -1492.7138)
  arc A12 (57.6984, -1659.0861) -> (-75.9333, -1492.7138) centre (-106.211, -1653.8864) ccw
  line L1 (57.7033, -1659.086) -> (57.7033, -1984.2902)
  arc A13 (-228.6216, -1991.6476) -> (57.7033, -1984.2902) centre (-85.5537, -1984.2902) ccw
  arc A14 (57.6986, -1648.6916) -> (1344.0583, -1343.2516) centre (-257.4199, 2539.899) ccw
  line L2 (1452.7286, 973.6047) -> (1452.7286, -1108.9917)
  arc A15 (1452.7286, -1108.9917) -> (1344.0583, -1343.2516) centre (1516.2092, -1280.775) ccw
  line L3 (1610.4916, -1203.7051) -> (1610.4916, -1659.0893)
  arc A16 (1344.0583, -1659.1876) -> (1610.4916, -1659.0893) centre (1477.2462, -1581.2147) ccw
  arc A17 (1610.4916, -1203.7051) -> (1452.7286, -1108.9917) centre (1452.3974, -1288.2919) ccw
  line L4 (1344.0583, -1343.2516) -> (1344.0583, -1659.1876)
  arc A18 (1610.4916, -1501.1715) -> (1905.3764, -933.777) centre (1179.1232, -916.6562) ccw
  line L5 (1834.9513, 1293.6308) -> (1834.9513, -822.26)
  line L6 (-228.6747, -1990.5298) -> (-228.6747, -1622.85)
  arc A19 (-75.9333, -1492.7138) -> (-228.6747, -1622.85) centre (-73.0964, -1650.7482) ccw
  line L7 (-1673.2082, 972.8146) -> (-1628.5464, -1108.9903)
  arc A20 (-1504.1047, -1343.2516) -> (-1628.5464, -1108.9903) centre (-1680.9694, -1287.0208) ccw
  line L8 (-1504.1047, -1343.2516) -> (-1504.1047, -1650.7481)
  arc A21 (-1504.1047, -1343.2516) -> (-228.6747, -1622.85) centre (-182.336, 1637.3619) ccw
  line L9 (-2082.4405, 1731.2909) -> (-2098.725, 1402.2239)
  arc A22 (-1787.8938, -1650.7481) -> (-1504.1047, -1650.7481) centre (-1645.9992, -1574.5739) ccw
  arc A23 (-1628.5464, -1108.9903) -> (-1787.8938, -1254.3066) centre (-1631.8203, -1265.4251) ccw
  line L10 (-1787.8938, -1254.3066) -> (-1787.8938, -1650.7481)
  arc A24 (-2074.0868, -925.1108) -> (-1787.8938, -1452.5274) centre (-1341.436, -868.9081) ccw
  arc A25 (-2017.5358, -581.1146) -> (-1737.2534, -1149.8118) centre (-1389.4828, -624.9959) ccw
  line L11 (1903.0093, 1658.484) -> (1903.0093, 1387.7061)
  line L12 (1903.0093, 1387.7061) -> (1925.3848, 1422.0781)
  line L13 (-1787.8938, 1459.2764) -> (-1787.8938, 1129.3874)
  line L14 (-1492.3011, 1043.103) -> (-1492.3011, 1375.2536)
  line L15 (-209.5648, 904.9842) -> (-209.5648, 1248.2771)
  line L16 (57.6983, 904.9842) -> (57.6983, 1248.2769)
  line L17 (1344.037, 1069.6986) -> (1344.037, 1384.9498)
  line L18 (1610.4923, 1148.3247) -> (1610.4923, 1442.784)
  arc A26 (-1517.0706, -1671.083) -> (-228.6747, -1990.5298) centre (-373.7717, 182.1722) ccw
  line L19 (1905.3764, -616.637) -> (1905.3764, -933.777)
  line L20 (-2074.0868, -925.1108) -> (-2074.0868, -496.0843)
  line L21 (-2017.5358, -581.1146) -> (-2017.5358, 1312.7645)
  line L22 (-2074.0868, -496.0843) -> (-2017.5358, -274.3431)
  line L23 (1905.3764, -624.9959) -> (1905.3764, -482.8395)
  line L24 (1905.3764, -482.8395) -> (1834.9513, -295.6547)
  arc A27 (1544.6867, -1134.5669) -> (1834.9513, -822.26) centre (1402.5875, -711.4545) ccw
  arc A28 (-1492.3011, 1375.2536) -> (-1787.8938, 1459.2764) centre (-1648.7566, 1386.8019) ccw
  arc A29 (-1492.3011, 1375.2536) -> (-209.5648, 1248.2771) centre (-326.4585, 6610.0874) ccw
  line L25 (-2082.4405, 1731.2909) -> (-2045.8113, 1840.8288) construction
  line L26 (-2045.8113, 1840.8288) -> (-1912.5822, 1937.0721) construction
  line L27 (-1912.5822, 1937.0721) -> (-1787.8938, 2044.1679) construction
  line L28 (-1787.8938, 2044.1679) -> (-1517.0706, 2107.2739) construction
  line L29 (-1517.0706, 2107.2739) -> (-1232.6657, 2183.169) construction
  line L30 (-1232.6657, 2183.169) -> (-897.8073, 2228.9905) construction
  line L31 (-897.8073, 2228.9905) -> (-602.5529, 2228.9905) construction
  line L32 (-602.5529, 2228.9905) -> (-209.5648, 2272.1913) construction
  line L33 (-209.5648, 2272.1913) -> (20.9738, 2272.1913) construction
  line L34 (20.9738, 2272.1913) -> (792.7366, 2205.1699) construction
  line L35 (792.7366, 2205.1699) -> (1344.037, 2107.2739) construction
  line L36 (1344.037, 2107.2739) -> (1609.3312, 2039.6154) construction
  line L37 (1609.3312, 2039.6154) -> (1794.4641, 1916.124) construction
  line L38 (1794.4641, 1916.124) -> (1925.3848, 1767.0325) construction
  line L39 (1925.3848, 1767.0325) -> (1903.0093, 1658.484) construction
  spline S0 degree 4 poles (-2082.4405, 1731.2909) (-2045.8113, 1840.8288) (-1912.5822, 1937.0721) (-1787.8938, 2044.1679) (-1517.0706, 2107.2739) (-1232.6657, 2183.169) (-897.8073, 2228.9905) (-602.5529, 2228.9905) (-209.5648, 2272.1913) (20.9738, 2272.1913) (792.7366, 2205.1699) (1344.037, 2107.2739) (1609.3312, 2039.6154) (1794.4641, 1916.124) (1925.3848, 1767.0325) (1903.0093, 1658.484) knots 1 1 1 1 1 2 3 4 5 6 7 8 9 10 11 12 13 13 13 13 13
  arc A30 (35.3855, 2263.9218) -> (-209.5648, 2265.0695) centre (-87.13, 2255.8862) ccw
  arc A31 (1602.9869, 2020.3473) -> (1344.037, 2100.6173) centre (1471.9332, 2055.3893) ccw
  arc A32 (57.7033, -1984.2902) -> (1344.0583, -1659.1876) centre (131.3506, 431.759) ccw
  arc A33 (-1517.0706, 2107.2739) -> (-1782.3432, 2020.3473) centre (-1644.0171, 2046.447) ccw
  point P0 (0, 0)
  point P1 (-1782.3432, 2020.3473)
  constraints: 80 point on circle, 50 end point, 34 centre point, 14 vertical, 6 parallel, 4 point on line, 2 horizontal, 1 coincident, 1 midpoint, 1 tangent, 12 other